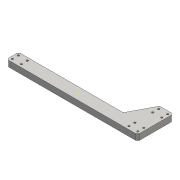
# Autodesk Inventor part: HorizontalBridge
Saved by Autodesk Inventor 2016 (Build 200138000, 138)
## iProperties
Created: 2016-12-22
Part Number: HorizontalBridge
Material: Generic
Document SubType Name: Modeling
Designer: inorn
Density: 1 g/cm^3
Appearance: Default
Author: inorn
Autodesk Inventor part; units mm, degrees
ref_plane "YZ Plane" through (0, 0, 0) normal (1, 0, 0) x (0, 1, 0)
ref_plane "XZ Plane" through (0, 0, 0) normal (0, 1, 0) x (-1, 0, 0)
ref_plane "XY Plane" through (0, 0, 0) normal (0, 0, 1) x (1, 0, 0)
sketch "Sketch1" plane through (0, 0, 0) normal (0, 0, 1) x (1, 0, 0)
  line L0 (-109.7639, -7) -> (-109.7639, 7)
  line L1 (-105.2639, 5) -> (-90.2639, 5) construction
  line L2 (-90.2639, 5) -> (-90.2639, -5) construction
  line L3 (-90.2639, -5) -> (-105.2639, -5) construction
  line L4 (-105.2639, -5) -> (-105.2639, 5) construction
  line L5 (-105.2639, 5) -> (-90.2639, -5) construction
  line L6 (-90.2639, 5) -> (-105.2639, -5) construction
  circle A0 centre (-105.2639, 5) radius 1.6
  circle A1 centre (-90.2639, 5) radius 1.6
  circle A2 centre (-105.2639, -5) radius 1.6
  circle A3 centre (-90.2639, -5) radius 1.6
  circle A4 centre (90.7361, 45) radius 1.6
  circle A5 centre (105.7361, 45) radius 1.6
  circle A6 centre (90.7361, 35) radius 1.6
  circle A7 centre (105.7361, 35) radius 1.6
  line L7 (-109.7639, 7) -> (-106.7639, 10)
  line L8 (-109.7639, -7) -> (-106.7639, -10)
  line L9 (87.2361, 50) -> (107.2361, 50)
  line L10 (110.2361, 47) -> (110.2361, -7)
  line L11 (107.2361, -10) -> (87.1625, -10)
  circle A8 centre (105.7361, -5) radius 1.6
  circle A9 centre (105.7361, 5) radius 1.6
  circle A10 centre (90.7361, -5) radius 1.6
  circle A11 centre (90.7361, 5) radius 1.6
  line L12 (90.7361, 45) -> (105.7361, 45) construction
  line L13 (105.7361, 35) -> (105.7361, 5) construction
  line L14 (107.2361, 50) -> (110.2361, 47)
  line L15 (110.2361, -7) -> (107.2361, -10)
  line L16 (87.2361, 50) -> (66.2361, 10)
  line L17 (87.1625, -10) -> (66, -10)
  line L18 (-106.7639, 10) -> (66.2361, 10)
  line L19 (66, -10) -> (-106.7639, -10)
  point P0 (0, 0)
  point P1 (0.2361, 0)
  point P2 (98.4723, 19.4096)
  point P3 (-97.7639, 0)
  point P4 (0.2361, 0)
  point P5 (98.2361, 45)
  point P6 (105.7361, 20)
  point P7 (98.2361, 20)
  dimension "d4" = 15
  dimension "d5" = 10
  dimension "d6" = 12
  dimension "d8" = 3.2
  dimension "d20" = 15
  dimension "d21" = 10
  dimension "d22" = 15
  dimension "d23" = 10
  dimension "d24" = 30
  dimension "d31" = 4.5
  dimension "d32" = 5
  dimension "d34" = 220
  dimension "d35" = 3
  dimension "d36" = 3
  dimension "d37" = 3
  dimension "d38" = 3
  dimension "d39" = 20
  constraints: 40 end point, 12 centre point, 7 equal radius, 6 parallel, 6 vertical alignment, 5 horizontal, 4 coincident, 4 horizontal alignment, 4 midpoint, 4 perpendicular, 1 vertical
  measures "d4" distance of L2.end L4.start
  measures "d5" distance of L6.start L2.end
  measures "d6" distance from line of point (-97.764, 0) L0
  measures "d8" diameter of A0
  measures "d20" distance of L12.end L12.start
  measures "d21" distance of L13.start L12.end
  measures "d22" distance of L13.end A11.centre
  measures "d23" distance of A8.centre L13.end
  measures "d24" distance of L13.end L13.start
  measures "d31" distance from line of L10 L12.end
  measures "d32" distance from line of L9 L12.end
  measures "d34" distance between parallel lines of L10 L0
  measures "d35" horizontal distance of L7.end L7.start
  measures "d36" horizontal distance of L7.end L7.start
  measures "d37" horizontal distance of L8.end L8.start
  measures "d38" horizontal distance of L8.start L8.end
  measures "d39" distance of L9.start L9.end
extrude "Extrusion1" add sketch "Sketch1" along normal blind 10
sketch "Sketch3" plane through (0, 0, 10) normal (0, 0, 1) x (1, 0, 0)
  point P0 (0, 0)
body "Solid1"
